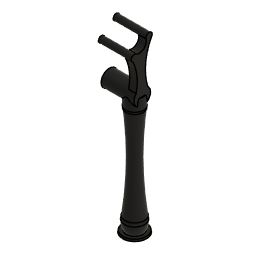
Laptop Stand (Autodesk Fusion 360 design; units mm, degrees)
Autodesk Fusion 360 part; units mm, degrees
sketch "Sketch1" plane through (0, 0, 0) normal (0, 0, 1) x (1, 0, 0)
  line L0 (139.7, -76.2) -> (-139.7, -76.2)
  line L1 (-139.7, -76.2) -> (-139.7, 76.2)
  line L2 (-139.7, 76.2) -> (139.7, 76.2)
  line L3 (139.7, 76.2) -> (139.7, -76.2)
  line L4 (139.7, -76.2) -> (-139.7, 76.2) construction
  line L5 (-139.7, -76.2) -> (139.7, 76.2) construction
  constraint horizontal L0
  constraint perpendicular L0 L1
  constraint parallel L0 L2
  constraint parallel L1 L3
  constraint coincident L4 origin
  constraint coincident L5 origin
extrude "Extrude1" add sketch "Sketch1" along normal blind 20.066 makes body 1
sketch "Sketch2" plane through (0, 0, 20.066) normal (0, 0, 1) x (-1, 0, 0)
  line L0 (-139.7, -76.2) -> (139.7, -76.2)
  line L1 (139.7, -76.2) -> (139.7, 76.2)
  line L2 (139.7, 76.2) -> (-139.7, 76.2)
  line L3 (-139.7, 76.2) -> (-139.7, -76.2)
  line L4 (-139.7, -63.4892) -> (139.7, -63.4892)
  line L5 (139.7, -63.4892) -> (139.7, -57.3932)
  line L6 (139.7, -57.3932) -> (-139.7, -57.3932)
  line L7 (-139.7, -57.3932) -> (-139.7, -63.4892)
  dimension "d5" = 6.096
  constraint horizontal L4
  constraint vertical L5
  constraint horizontal L6
  constraint vertical L7
  constraint coincident L1 L5.end
  constraint coincident L3 L4.start
  measures "d5" distance of L4 L6
extrude "Extrude2" add sketch "Sketch2" along normal blind 190.5 separate body contours L1 L3 L4 L5 L6 L7 makes body 2
move_body "Move1" bodies 1 to x (1, 0, 0) y (0, 0.766044, 0.642788) z (0, -0.642788, 0.766044) at (0, 36.051, -15.2294)
extrude "Extrude3" add 1 faces at (46.5667, -26.6209, -59.086) along direction (0, -0.766044, -0.642788) blind 63.5 on bodies 1 bodies 1
sketch "Sketch3" plane through (139.7, 0, 0) normal (1, 0, 0) x (0, 1, 0)
  line L0 (-70.9654, -105.0269) -> (94.4236, 33.751)
  line L1 (94.4236, 33.751) -> (81.5255, 49.1224)
  line L2 (81.5255, 49.1224) -> (-83.8635, -89.6554)
  line L3 (-83.8635, -89.6554) -> (-70.9654, -105.0269)
  circle A0 centre (67.5796, 41.5294) radius 3.175
  circle A1 centre (52.7518, 29.6028) radius 3.175
  arc A2 (54.9525, 31.8915) -> (64.619, 40.3823) centre (57.722, 38.4864) ccw
  line L4 (67.5796, 41.5294) -> (70.7546, 41.5294) construction
  circle A3 centre (60.682, -8.0021) radius 8.3433
  arc A4 (54.5367, -2.3589) -> (51.3592, 26.7495) centre (11.9299, 7.7179) ccw
  arc A5 (69.9212, 39.3853) -> (66.2504, -1.7888) centre (118.8544, 14.272) ccw
  line L5 (50.6095, -129.5141) -> (70.7546, -129.5141)
  dimension "d8" = 6.35
  dimension "d9" = 6.35
  constraint tangent L2 A2
  constraint coincident A0 A2.end
  constraint coincident A1 A2.start
  constraint coincident A0.centre L4.start
  constraint coincident A0 L4.end
  constraint horizontal L4
  constraint coincident A3 A4.start
  constraint coincident A1 A4.end
  constraint coincident A0 A5.start
  constraint coincident L2 A5.start
  constraint coincident A3 A5.end
  measures "d8" diameter of A0
  measures "d9" diameter of A1
extrude "Extrude4" add 1 faces at (46.5667, -75.2648, -99.903) along direction (0, -0.766044, -0.642788) blind 43.942 on bodies 1 bodies 1
extrude "Extrude5" add sketch "Sketch3" against normal blind 25.4 separate body contours A3 | L2 A0 | A1 picked at (66.6047, 41.8239) makes body 3 at (122.7667, 55.9111, 29.2867) makes body 4 at (131.2333, 69.4958, 44.0609) makes body 5 at (122.7667, 68.9839, -8.8328)
extrude "Extrude6" add sketch "Sketch3" along normal blind 7.62 separate body contours L0 L2 A0 A4 A5 | L0 A3 A4 A5 | A3 | L2 A1 A2 A4 | L2 A0 | L2 A0 A2 | A1 picked at (66.6047, 41.8239) makes body 6
sketch "Sketch4" plane through (139.7, 0, 0) normal (1, 0, 0) x (0, 1, 0)
  line L0 (60.682, -8.002) -> (60.682, -129.54)
  line L1 (60.682, -8.002) -> (69.0215, -8.002) construction
  line L2 (69.0215, -129.54) -> (60.682, -129.54)
  line L3 (69.0215, -129.54) -> (76.2, -129.54)
  line L4 (76.2, -129.54) -> (76.2, -127.7087)
  line L5 (76.2, -127.7087) -> (69.0215, -127.7087)
  line L6 (69.0215, -8.002) -> (60.682, -8.002)
  line L7 (69.0215, -8.002) -> (69.0215, -12.6531) construction
  arc A0 (69.0215, -127.7087) -> (70.8189, -118.1454) centre (50.7285, -119.32) ccw
  arc A1 (69.6055, -19.2012) -> (69.0215, -8.002) centre (29.7954, -15.6622) ccw
  arc A2 (69.3823, -21.269) -> (70.4395, -114.9343) centre (447.9972, -63.8345) ccw
  arc A3 (72.3895, -127.7087) -> (72.7055, -129.54) centre (447.9972, -63.8345) ccw
  arc A4 (70.4395, -114.9343) -> (70.8868, -118.1373) centre (70.6597, -116.5363) ccw
  arc A5 (69.6055, -19.2012) -> (69.3823, -21.269) centre (69.4999, -20.2358) ccw
  dimension "d22" = 762
  constraint vertical L0
  constraint perpendicular L0 L1
  constraint perpendicular L1 L7
  constraint perpendicular L0 L2
  constraint perpendicular L3 L7
  constraint perpendicular L3 L4
  constraint coincident L5.end L7
  constraint perpendicular L5 L7
  constraint tangent A0 A2
  constraint tangent A1 A2
  constraint coincident L3 A3.end
  constraint coincident L5 A3.start
  constraint concentric A2 A3
  constraint coincident A4 A0.end
  measures "d22" diameter of A2
revolve "Revolve1" add sketch "Sketch4" angle 360 about axis through (139.7, 60.682, -8.002) along (0, 0, -1) separate body contours L0 L2 L3 L5 L6 A0 A1 A2 A3 A4 A5 makes body 7
combine "Combine1" operation add target body 6 tool bodies 3 4 5 7
hidden bodies 1 2
equation "d11 = 10.23 in - 8.5 in"
